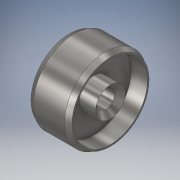
# Autodesk Inventor part: wheel
Saved by Autodesk Inventor 2019 (Build 230136000, 136)
## iProperties
Created: 2021-06-13
Part Number: wheel
Material: Iron, Malleable
Document SubType Name: Modeling
Designer: joelm
Density: 7.15 g/cm^3
Appearance: Semi-Polished
Author: joelm
Autodesk Inventor part; units mm, degrees
ref_plane "YZ Plane" through (0, 0, 0) normal (1, 0, 0) x (0, 1, 0)
ref_plane "XZ Plane" through (0, 0, 0) normal (0, 1, 0) x (-1, 0, 0)
ref_plane "XY Plane" through (0, 0, 0) normal (0, 0, 1) x (1, 0, 0)
sketch "Sketch1" plane through (0, 0, 0) normal (0, 0, 1) x (1, 0, 0)
  line L0 (0, 0) -> (50, 0)
  line L1 (6, 11) -> (44, 11)
  line L2 (6, 50) -> (44, 50)
  line L3 (0, 45) -> (0, 47)
  line L4 (50, 45) -> (50, 47)
  line L5 (0, 47) -> (6, 50)
  line L6 (44, 50) -> (50, 47)
  line L7 (20, 18) -> (20, 45)
  line L8 (30, 18) -> (30, 45)
  line L9 (6, 11) -> (0, 18)
  line L10 (44, 11) -> (50, 18)
  line L11 (0, 45) -> (20, 45)
  line L12 (30, 45) -> (50, 45)
  line L13 (0, 18) -> (20, 18)
  line L14 (30, 18) -> (50, 18)
  dimension "d0" = 50
  dimension "d2" = 38
  dimension "d3" = 11
  dimension "d4" = 39
  dimension "d6" = 2
  dimension "d7" = 2
  dimension "d8" = 10
  dimension "d9" = 20
  constraints: 30 end point, 8 parallel, 2 horizontal, 2 perpendicular, 2 vertical
  measures "d0" distance of L0.start L0.end
  measures "d2" distance of L1.start L1.end
  measures "d3" vertical distance of L1.start L0.start
  measures "d4" distance between parallel lines of L1 L2
  measures "d6" distance of L3.start L3.end
  measures "d7" distance of L4.start L4.end
  measures "d8" distance between parallel lines of L7 L8
  measures "d9" distance from line of L7 L0.start
revolve "Revolution1" add sketch "Sketch1" angle 360 about axis through (0, 0, 0) along (1, 0, 0)
body "Solid1"
